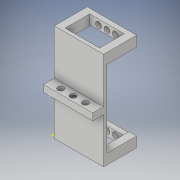
# Autodesk Inventor part: Objektträgerhalter 1.1 final
Saved by Autodesk Inventor 2018.3 (Build 223284000, 284)
## iProperties
Created: 2018-11-22
Part Number: Objektträgerhalter 1.1 final
Material: Generisch
Document SubType Name: Modeling
Designer: pgmadmin
Density: 1 g/cm^3
Appearance: Vorgabe
Author: pgmadmin
Autodesk Inventor part; units mm, degrees
ref_plane "YZ Plane" through (0, 0, 0) normal (1, 0, 0) x (0, 1, 0)
ref_plane "XZ Plane" through (0, 0, 0) normal (0, 1, 0) x (-1, 0, 0)
ref_plane "XY Plane" through (0, 0, 0) normal (0, 0, 1) x (1, 0, 0)
sketch "Skizze1" plane through (0, 0, 0) normal (0, 0, 1) x (1, 0, 0)
  line L0 (-6.5297, -2.8796) -> (43.4703, -2.8796)
  line L1 (43.4703, -2.8796) -> (43.4703, 8.1204)
  line L2 (43.4703, 8.1204) -> (-6.5297, 8.1204)
  line L3 (-6.5297, 8.1204) -> (-6.5297, -2.8796)
  point P0 (0, 0)
  dimension "d0" = 50
  dimension "d1" = 11
  constraints: 8 end point, 2 parallel, 1 horizontal, 1 perpendicular
  measures "d0" distance of L2.end L1.end
  measures "d1" distance of L1.end L0.end
extrude "Extrusion1" add sketch "Skizze1" along normal blind 7
sketch "Skizze2" plane through (-6.5297, 8.1204, 0) normal (0, 1, 0) x (1, 0, 0)
  line L0 (29.65, -5.55) -> (20.35, -5.55)
  line L1 (20.35, -5.55) -> (20.35, -1.45)
  line L2 (20.35, -1.45) -> (29.65, -1.45)
  line L3 (29.65, -1.45) -> (29.65, -5.55)
  line L4 (50, -7) -> (0, -7) projected
  line L5 (50, 0) -> (50, -7) projected
  line L6 (0, 0) -> (0, -7) projected
  point P0 (6.5297, 0)
  dimension "d4" = 9.3
  dimension "d5" = 4.1
  dimension "d6" = 1.45
  dimension "d7" = 20.35
  dimension "d8" = 20.35
  constraints: 8 end point, 2 parallel, 1 horizontal, 1 perpendicular
  measures "d4" distance of L1.end L2.end
  measures "d5" distance of L0.end L1.end
  measures "d6" distance between parallel lines of L4 L0
  measures "d7" distance between parallel lines of L5 L3
  measures "d8" distance between parallel lines of L1 L6
extrude "Extrusion2" cut sketch "Skizze2" against normal blind 9.35
sketch "Skizze3" plane through (0, 0, 7) normal (0, 0, 1) x (1, 0, 0)
  line L0 (-6.5297, 8.1204) -> (-6.5297, -2.8796) projected
  line L1 (43.4703, 8.1204) -> (-6.5297, 8.1204) projected
  point P0 (0, 0)
  point P1 (5.9703, 2.2704)
  point P2 (18.4703, 2.2704)
  point P3 (30.9703, 2.2704)
  dimension "d11" = 12.5
  dimension "d12" = 12.5
  dimension "d13" = 12.5
  dimension "d14" = 5.85
  measures "d11" distance from line of L0 point (5.97, 2.27)
  measures "d12" distance of point (5.97, 2.27) point (18.47, 2.27)
  measures "d13" distance of point (30.97, 2.27) point (18.47, 2.27)
  measures "d14" distance from line of L1 point (5.97, 2.27)
hole "Bohrung1" at (5.9703, 2.2704, 7) at (18.4703, 2.2704, 7) at (30.9703, 2.2704, 7) direction (0, 0, -1) diameter 6.15 end through all
sketch "Skizze4" plane through (-6.5297, 8.1204, 0) normal (0, 1, 0) x (1, 0, 0)
  point P0 (6.5297, 0)
sketch "Skizze5" plane through (-6.5297, 8.1204, 0) normal (0, 1, 0) x (1, 0, 0)
  line L0 (50, 0) -> (0, 0) projected
  line L1 (0, 0) -> (0, -53.0037)
  line L2 (0, -53) -> (50, -53)
  line L3 (50, -53) -> (50, 46)
  line L4 (50, 46) -> (0, 46)
  line L5 (0, 46) -> (0, -53)
  point P0 (6.5297, 0)
  dimension "d22" = 50
  dimension "d23" = 99
  dimension "d24" = 46
  constraints: 10 end point, 2 parallel, 1 horizontal, 1 perpendicular, 1 point on line, 1 vertical
  measures "d22" distance of L4.end L3.end
  measures "d23" distance of L3.end L2.end
  measures "d24" distance between parallel lines of L4 L0
extrude "Extrusion3" add sketch "Skizze5" along normal blind 3.5
sketch "Skizze6" plane through (-6.5297, 11.6204, 0) normal (0, 1, 0) x (1, 0, 0)
  line L0 (29.65, -1.45) -> (29.65, -5.55) projected
  line L1 (29.65, -1.45) -> (20.35, -1.45)
  line L2 (20.35, -1.45) -> (20.35, -5.55)
  line L3 (20.35, -5.55) -> (29.65, -5.55)
  line L4 (29.65, -5.55) -> (29.65, -1.45)
  point P0 (6.5297, 0)
  constraints: 8 end point, 2 parallel, 1 horizontal, 1 perpendicular
extrude "Extrusion4" cut sketch "Skizze6" against normal blind 3.5
sketch "Skizze7" plane through (-6.5297, 11.6204, 0) normal (0, 1, 0) x (1, 0, 0)
  line L0 (0, -53) -> (50, -53) projected
  line L1 (50, -53) -> (42.5, -53)
  line L2 (42.5, -53) -> (42.5, -42.5)
  line L3 (42.5, -42.5) -> (50, -42.5)
  line L4 (50, -42.5) -> (50, -53)
  line L5 (0, -53) -> (7.5, -53)
  line L6 (7.5, -53) -> (7.5, -42.5)
  line L7 (7.5, -42.5) -> (0, -42.5)
  line L8 (0, -42.5) -> (0, -53)
  line L9 (0, 46) -> (0, -53) projected
  line L10 (0, 46) -> (7.5, 46)
  line L11 (7.5, 46) -> (7.5, 35.5)
  line L12 (7.5, 35.5) -> (0, 35.5)
  line L13 (0, 35.5) -> (0, 46)
  line L14 (50, -53) -> (50, 46) projected
  line L15 (50, 46) -> (42.5, 46)
  line L16 (42.5, 46) -> (42.5, 35.5)
  line L17 (42.5, 35.5) -> (50, 35.5)
  line L18 (50, 35.5) -> (50, 46)
  point P0 (6.5297, 0)
  dimension "d29" = 7.5
  dimension "d30" = 10.5
  dimension "d31" = 7.5
  dimension "d32" = 10.5
  dimension "d33" = 7.5
  dimension "d34" = 10.5
  dimension "d35" = 7.5
  dimension "d36" = 10.5
  constraints: 32 end point, 8 parallel, 4 horizontal, 4 perpendicular
  measures "d29" distance of L2.end L3.end
  measures "d30" distance of L1.end L2.end
  measures "d31" distance of L7.end L6.end
  measures "d32" distance of L6.end L5.end
  measures "d33" distance of L11.end L12.end
  measures "d34" distance of L10.end L11.end
  measures "d35" distance of L17.end L16.end
  measures "d36" distance of L16.end L15.end
extrude "Extrusion5" add sketch "Skizze7" along normal blind 25
sketch "Skizze8" plane through (0.9703, 11.6204, -35.5) normal (1, 0, 0) x (0, 0, -1)
  point P0 (-35.5, -11.6204)
sketch "Skizze9" plane through (-6.5297, 36.6204, 0) normal (0, 1, 0) x (1, 0, 0)
  line L0 (50, -42.5) -> (50, 35.5) projected
  line L1 (0, 46) -> (50, 46)
  line L2 (50, 46) -> (50, 35.5)
  line L3 (50, 35.5) -> (0, 35.5)
  line L4 (0, 35.5) -> (0, 46)
  line L5 (50, -53) -> (50, -7) projected
  line L6 (0, -42.5) -> (50, -42.5)
  line L7 (50, -42.5) -> (50, -53)
  line L8 (50, -53) -> (0, -53)
  line L9 (0, -53) -> (0, -42.5)
  line L10 (50, -42.5) -> (42.5, -42.5) projected
  point P0 (6.5297, 0)
  dimension "d75" = 0
  constraints: 16 end point, 4 parallel, 2 horizontal, 2 perpendicular, 1 point on line
  measures "d75" distance between parallel lines of L6 L10
extrude "Extrusion6" add sketch "Skizze9" along normal blind 5
sketch "Skizze10" plane through (-6.5297, 41.6204, 0) normal (0, 1, 0) x (1, 0, 0)
  line L0 (50, 46) -> (0, 46) projected
  line L1 (0, -53) -> (50, -53) projected
  line L2 (42.5, -42.5) -> (42.5, -53) projected
  line L3 (42.5, 46) -> (42.5, 35.5) projected
  line L4 (7.5, 35.5) -> (7.5, 46) projected
  line L5 (7.5, -53) -> (7.5, -42.5) projected
  point P0 (6.5297, 0)
  point P1 (15.7518, 40.75)
  point P2 (25, 40.75)
  point P3 (33.5, 40.75)
  point P4 (15.6745, -47.75)
  point P5 (25, -47.75)
  point P6 (33.5, -47.75)
  dimension "d41" = 5.25
  dimension "d42" = 5.25
  dimension "d43" = 5.25
  dimension "d44" = 5.25
  dimension "d45" = 5.25
  dimension "d46" = 5.25
  dimension "d47" = 9
  dimension "d50" = 9
  dimension "d76" = 17.5
  dimension "d77" = 17.5
  measures "d41" distance from line of L0 point (33.5, 40.75)
  measures "d42" distance from line of L0 point (25, 40.75)
  measures "d43" distance from line of L0 point (15.752, 40.75)
  measures "d44" distance from line of L1 point (15.674, -47.75)
  measures "d45" distance from line of L1 point (25, -47.75)
  measures "d46" distance from line of L1 point (33.5, -47.75)
  measures "d47" distance from line of L2 point (33.5, -47.75)
  measures "d50" distance from line of L3 point (33.5, 40.75)
  measures "d76" distance from line of L4 point (25, 40.75)
  measures "d77" distance from line of L5 point (25, -47.75)
hole "Bohrung2" at (18.4703, 41.6204, 47.75) at (18.4703, 41.6204, -40.75) direction (0, -1, 0) diameter 6 depth 10 tip angle 118
sketch "Skizze11" plane through (-6.5297, 41.6204, 0) normal (0, 1, 0) x (1, 0, 0)
  line L0 (7.5, -53) -> (7.5, -42.5) projected
  line L1 (42.5, -42.5) -> (42.5, -53) projected
  line L2 (50, -42.5) -> (0, -42.5) projected
  line L3 (50, 46) -> (0, 46) projected
  line L4 (42.5, 46) -> (42.5, 35.5) projected
  line L5 (7.5, 35.5) -> (7.5, 46) projected
  point P0 (6.5297, 0)
  point P1 (16.5, -47.75)
  point P2 (33.5, -47.75)
  point P3 (16.5, 40.75)
  point P4 (33.5, 40.75)
  dimension "d60" = 9
  dimension "d61" = 9
  dimension "d62" = 5.25
  dimension "d63" = 5.25
  dimension "d64" = 5.25
  dimension "d65" = 5.25
  dimension "d66" = 9
  dimension "d67" = 9
  measures "d60" distance from line of L0 point (16.5, -47.75)
  measures "d61" distance from line of L1 point (33.5, -47.75)
  measures "d62" distance from line of L2 point (16.5, -47.75)
  measures "d63" distance from line of L2 point (33.5, -47.75)
  measures "d64" distance from line of L3 point (16.5, 40.75)
  measures "d65" distance from line of L3 point (33.5, 40.75)
  measures "d66" distance from line of L4 point (33.5, 40.75)
  measures "d67" distance from line of L5 point (16.5, 40.75)
hole "Bohrung3" at (9.9703, 41.6204, 47.75) at (26.9703, 41.6204, 47.75) at (9.9703, 41.6204, -40.75) at (26.9703, 41.6204, -40.75) direction (0, -1, 0) diameter 6.2 depth 31.5 tip angle 118
sketch "Skizze12" plane through (-6.5297, -2.8796, 0) normal (0, -1, 0) x (1, 0, 0)
  point P0 (6.5297, 0)
sketch "Skizze13" plane through (-6.5297, 41.6204, 0) normal (0, 1, 0) x (1, 0, 0)
  line L0 (42.5, -53) -> (42.5, -42.5) projected
  line L1 (7.5, -42.5) -> (7.5, -53) projected
  line L2 (42.5, -42.5) -> (7.5, -42.5)
  line L3 (7.5, -42.5) -> (7.5, -43.46)
  line L4 (7.5, -43.46) -> (42.5, -43.46)
  line L5 (42.5, -43.46) -> (42.5, -42.5)
  point P0 (6.5297, 0)
  dimension "d78" = 0.96
  constraints: 8 end point, 2 parallel, 1 horizontal, 1 perpendicular, 1 point on line
  measures "d78" distance between parallel lines of L4 L2
extrude "Extrusion7" cut sketch "Skizze13" against normal blind 10
sketch "Skizze14" plane through (35.9703, 11.6204, -35.5) normal (0, 0, 1) x (1, 0, 0)
  point P0 (-35.9703, -11.6204)
sketch "Skizze15" plane through (-6.5297, 41.6204, 0) normal (0, 1, 0) x (1, 0, 0)
  line L0 (7.5, 46) -> (7.5, 35.5) projected
  line L1 (42.5, 35.5) -> (7.5, 35.5)
  line L2 (7.5, 35.5) -> (7.5, 36.48)
  line L3 (7.5, 36.48) -> (42.5, 36.48)
  line L4 (42.5, 36.48) -> (42.5, 35.5)
  line L5 (0, 35.5) -> (50, 35.5) projected
  point P0 (6.5297, 0)
  dimension "d81" = 0.98
  dimension "d82" = 0
  constraints: 8 end point, 2 parallel, 1 horizontal, 1 perpendicular, 1 point on line
  measures "d81" distance between parallel lines of L1 L3
  measures "d82" distance between parallel lines of L5 L1
extrude "Extrusion8" cut sketch "Skizze15" against normal blind 10
